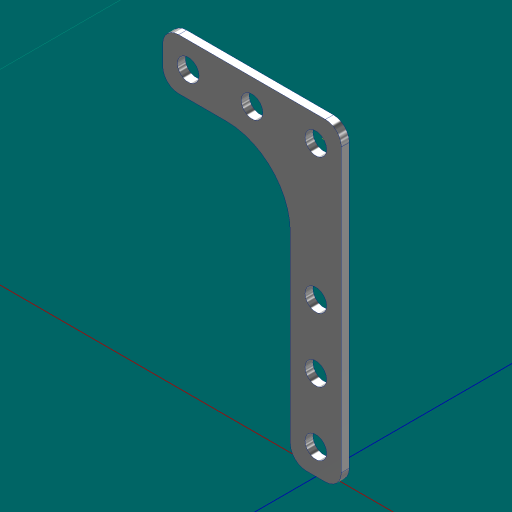
# Autodesk Inventor part: Inner_Strut_Gusset
Saved by Autodesk Inventor 2023.1 (Build 271208000, 208)
## iProperties
Created: 2022-11-06
Part Number: Inner_Strut_Gusset
Material: Aluminum 6061
Document SubType Name: Modeling
Designer: zac-h
Density: 2.7 g/cm^3
Appearance: Aluminum - Flat
Author: zac-h
Autodesk Inventor part; units mm, degrees
ref_plane "YZ Plane" through (0, 0, 0) normal (1, 0, 0) x (0, 1, 0)
ref_plane "XZ Plane" through (0, 0, 0) normal (0, 1, 0) x (-1, 0, 0)
ref_plane "XY Plane" through (0, 0, 0) normal (0, 0, 1) x (1, 0, 0)
sketch "Sketch1" plane through (0, 0, 0) normal (0, 0, 1) x (1, 0, 0)
  circle A0 centre (0, 0) radius 2.159
  line L0 (0, 0) -> (-38.1, 0) construction
  line L1 (0, 0) -> (0, -26.9418) construction
  circle A1 centre (-12.7, 0) radius 2.159
  circle A2 centre (-25.4, 0) radius 2.159
  circle A3 centre (0, -26.9418) radius 2.159
  circle A4 centre (0, -39.6418) radius 2.159
  circle A5 centre (0, -52.3418) radius 2.159
  line L2 (5.08, -57.4218) -> (-5.08, -57.4218)
  line L3 (-5.08, -57.4218) -> (-5.08, 5.08)
  line L4 (-5.08, 5.08) -> (5.08, 5.08)
  line L5 (5.08, 5.08) -> (5.08, -57.4218)
  circle A6 centre (0, -52.3418) radius 5.08 construction
  circle A7 centre (0, 0) radius 5.08 construction
  line L6 (5.08, 5.08) -> (-30.48, 5.08)
  line L7 (-30.48, 5.08) -> (-30.48, -5.08)
  line L8 (-30.48, -5.08) -> (5.08, -5.08)
  line L9 (5.08, -5.08) -> (5.08, 5.08)
  circle A8 centre (-25.4, 0) radius 5.08 construction
  point P0 (-5.08, 5.08)
  point P1 (-5.08, -5.08)
  point P2 (-5.08, 5.08)
  point P3 (5.08, -5.08)
  dimension "d5" = 12.7
  dimension "d21" = 26.9418
  dimension "d22" = 4.318
  dimension "d25" = 12.7
  dimension "d30" = 10.16
  constraints: 20 end point, 9 centre point, 8 tangent, 5 coincident, 4 horizontal, 4 parallel, 2 perpendicular, 2 vertical, 1 equal radius, 8 other
  measures "d5" distance of L0.start A1.centre
  measures "d21" distance of L0.start L1.end
  measures "d22" diameter of A0
  measures "d25" distance of A3.centre A4.centre
  measures "d30" diameter of A6
extrude "Extrusion1" add sketch "Sketch1" along normal blind 1.5875
fillet "Fillet1" radius 3.175 5 edges at (-30.48, -5.08, 0.7937) (-30.48, 5.08, 0.7937) (5.08, 5.08, 0.7937) (5.08, -57.4218, 0.7937) (-5.08, -57.4218, 0.7937)
fillet "Fillet2" radius 12.7 1 edges at (-5.08, -5.08, 0.7937)
body "Solid1"
